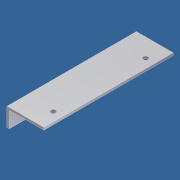
# Autodesk Inventor part: GE-12028-06
Saved by Autodesk Inventor 2012 (Build 160160000, 160)
## iProperties
Created: 2011-10-09
Part Number: GE-12028-06
Document SubType Name: Modeling
Designer: dfoster
Density: 1 g/cm^3
Description: Mounting Bracket, Chute
Material: Default
Title: Mounting Bracket, CHute
Author: dfoster
Autodesk Inventor part; units mm, degrees
ref_plane "YZ Plane" through (0, 0, 0) normal (1, 0, 0) x (0, 1, 0)
ref_plane "XZ Plane" through (0, 0, 0) normal (0, 1, 0) x (-1, 0, 0)
ref_plane "XY Plane" through (0, 0, 0) normal (0, 0, 1) x (1, 0, 0)
sketch "Sketch1" plane through (0, 0, 0) normal (0, 0, 1) x (1, 0, 0)
  line L0 (0, 0) -> (50.8, 0)
  line L1 (50.8, 0) -> (50.8, -3.175)
  line L2 (50.8, -3.175) -> (3.175, -3.175)
  line L3 (3.175, -3.175) -> (3.175, -25.4)
  line L4 (3.175, -25.4) -> (0, -25.4)
  line L5 (0, -25.4) -> (0, 0)
  dimension "d0" = 3.175
  dimension "d1" = 50.8
  dimension "d2" = 25.4
  constraints: 12 end point, 4 parallel, 2 perpendicular, 1 horizontal
  measures "d0" distance between parallel lines of L2 L0
  measures "d1" distance of L0.start L0.end
  measures "d2" distance of L4.end L0.start
extrude "Extrusion1" add sketch "Sketch1" along normal blind 177.8
hole "Hole1" at (38.1, 0, 152.4) direction (0, -1, 0) diameter 6.731 depth 25.4 tip angle 118
pattern_linear "Rectangular Pattern1" count 2 spacing 127 along (0, 0, -1) of "Hole1"
body "Solid1"
